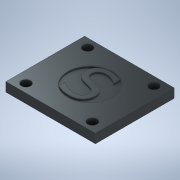
# Autodesk Inventor part: Part5
Saved by Autodesk Inventor 2020 (Build 240168000, 168)
## iProperties
Created: 2021-10-14
Part Number: Part5
Material: Iron, Cast
Document SubType Name: Modeling
Designer: simon.erikssonwestl
Density: 7.15 g/cm^3
Appearance: Iron Gray
Author: simon.erikssonwestl
Autodesk Inventor part; units mm, degrees
ref_plane "YZ Plane" through (0, 0, 0) normal (1, 0, 0) x (0, 1, 0)
ref_plane "XZ Plane" through (0, 0, 0) normal (0, 1, 0) x (-1, 0, 0)
ref_plane "XY Plane" through (0, 0, 0) normal (0, 0, 1) x (1, 0, 0)
sketch "Sketch1" plane through (0, 0, 0) normal (0, 1, 0) x (-1, 0, 0)
  line L0 (14.5, 12.75) -> (-14.5, 12.75)
  line L1 (-14.5, 12.75) -> (-14.5, -12.75)
  line L2 (-14.5, -12.75) -> (14.5, -12.75)
  line L3 (14.5, -12.75) -> (14.5, 12.75)
  line L4 (14.5, 12.75) -> (-14.5, -12.75) construction
  line L5 (-14.5, 12.75) -> (14.5, -12.75) construction
  point P0 (0, 0)
  dimension "d0" = 29
  dimension "d1" = 25.5
  constraints: 12 end point, 2 midpoint, 2 parallel, 1 horizontal, 1 perpendicular
  measures "d0" distance of L2.end L1.end
  measures "d1" distance of L1.end L0.end
extrude "Extrusion1" add sketch "Sketch1" along normal mid plane 3
sketch "Sketch2" plane through (0, 1.5, 0) normal (0, 1, 0) x (1, 0, 0)
  circle A0 centre (-10.75, 10) radius 1.5
  line L0 (14.5, 12.75) -> (-14.5, 12.75) projected
  line L1 (-14.5, 12.75) -> (-14.5, -12.75) projected
  circle A1 centre (10.75, 10) radius 1.5
  circle A2 centre (-10.75, -10) radius 1.5
  circle A3 centre (10.75, -10) radius 1.5
  point P0 (0, 0)
  dimension "d4" = 3
  dimension "d5" = 2.75
  dimension "d6" = 3.75
  dimension "d9" = 21.5
  dimension "d12" = 20
  constraints: 4 centre point, 1 horizontal, 1 vertical, 6 other
  measures "d4" diameter of A0
  measures "d5" distance from line of L0 A0.centre
  measures "d6" distance from line of L1 A0.centre
  measures "d9" distance of A0.centre A1.centre
  measures "d12" distance of A0.centre A2.centre
sketch "Sketch3" plane through (0, 1.5, 0) normal (0, 1, 0) x (1, 0, 0)
  circle A0 centre (0, 0) radius 7.25
  dimension "d15" = 14.5
  constraints: 1 centre point, 1 coincident
  measures "d15" diameter of A0
extrude "Extrusion2" cut sketch "Sketch2" against normal through all
sketch "Sketch4" plane through (0, 1.5, 0) normal (0, 1, 0) x (1, 0, 0)
  line L0 (-5.4078, 7.0301) -> (8.8628, 7.0301) construction
  line L1 (8.8628, 7.0301) -> (8.8628, -8.322) construction
  line L2 (8.8628, -8.322) -> (-5.4078, -8.322) construction
  line L3 (-5.4078, -8.322) -> (-5.4078, 7.0301) construction
  spline S0 degree 2 poles (-0.467, -6.4334) (-1.8786, -6.4334) (-3.8592, -5.8434) (-4.7336, -5.4221) knots 0 0 0 1 2 2 2
  line L4 (-4.7336, -5.4221) -> (-4.7336, -3.2519)
  line L5 (-4.7336, -3.2519) -> (-4.6072, -3.2519)
  spline S1 degree 2 poles (-4.6072, -3.2519) (-3.7538, -4.0525) (-1.5942, -4.9374) (-0.5934, -4.9374) knots 0 0 0 1 2 2 2
  spline S2 degree 2 poles (-0.5934, -4.9374) (0.8394, -4.9374) (2.3037, -3.747) (2.3037, -2.7673) knots 0 0 0 1 2 2 2
  spline S3 degree 2 poles (2.3037, -2.7673) (2.3037, -1.9877) (1.5347, -1.0185) (0.7024, -0.7762) knots 0 0 0 1 2 2 2
  spline S4 degree 2 poles (0.7024, -0.7762) (0.1019, -0.6076) (-0.8989, -0.3759) (-1.6469, -0.1862) knots 0 0 0 1 2 2 2
  spline S5 degree 2 poles (-1.6469, -0.1862) (-2.3211, -0.0071) (-3.3851, 0.5301) (-3.796, 0.9621) knots 0 0 0 1 2 2 2
  spline S6 degree 2 poles (-3.796, 0.9621) (-4.1963, 1.394) (-4.6388, 2.5528) (-4.6388, 3.3113) knots 0 0 0 1 2 2 2
  spline S7 degree 2 poles (-4.6388, 3.3113) (-4.6388, 4.8916) (-2.1736, 7.0301) (-0.2668, 7.0301) knots 0 0 0 1 2 2 2
  spline S8 degree 2 poles (-0.2668, 7.0301) (0.8288, 7.0301) (2.7672, 6.5982) (3.5995, 6.1873) knots 0 0 0 1 2 2 2
  line L6 (3.5995, 6.1873) -> (3.5995, 4.1225)
  line L7 (3.5995, 4.1225) -> (3.4731, 4.1225)
  spline S9 degree 2 poles (3.4731, 4.1225) (2.8515, 4.6914) (0.9131, 5.5342) (-0.1509, 5.5342) knots 0 0 0 1 2 2 2
  spline S10 degree 2 poles (-0.1509, 5.5342) (-1.3519, 5.5342) (-2.8373, 4.407) (-2.8373, 3.4904) knots 0 0 0 1 2 2 2
  spline S11 degree 2 poles (-2.8373, 3.4904) (-2.8373, 2.6687) (-1.9629, 1.689) (-1.1412, 1.4677) knots 0 0 0 1 2 2 2
  spline S12 degree 2 poles (-1.1412, 1.4677) (-0.5934, 1.3203) (0.9974, 0.941) (1.5241, 0.783) knots 0 0 0 1 2 2 2
  spline S13 degree 2 poles (1.5241, 0.783) (2.8621, 0.3721) (4.1052, -1.2819) (4.1052, -2.4934) knots 0 0 0 1 2 2 2
  spline S14 degree 2 poles (4.1052, -2.4934) (4.1052, -3.2624) (3.4836, -4.7373) (2.9253, -5.2535) knots 0 0 0 1 2 2 2
  spline S15 degree 2 poles (2.9253, -5.2535) (2.3037, -5.8224) (0.7235, -6.4334) (-0.467, -6.4334) knots 0 0 0 1 2 2 2
  point P0 (0, 0)
  constraints: 2 other
extrude "Extrusion3" cut sketch "Sketch3" against normal blind 0.5
extrude "Extrusion4" add sketch "Sketch4" against normal blind 0.5
body "Solid1"
